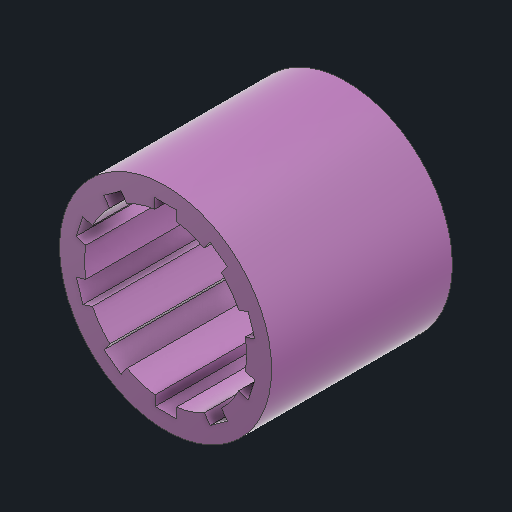
# Autodesk Inventor part: opona_CPY
Saved by Autodesk Inventor 2024 (Build 280153000, 153)
## iProperties
Created: 2024-05-24
Part Number: opona_CPY
Material: Generic
Document SubType Name: Modeling
Designer: Adam
Density: 1 g/cm^3
Appearance: Default
Author: Adam
Autodesk Inventor part; units mm, degrees
ref_plane "YZ Plane" through (0, 0, 0) normal (1, 0, 0) x (0, 1, 0)
ref_plane "XZ Plane" through (0, 0, 0) normal (0, 1, 0) x (-1, 0, 0)
ref_plane "XY Plane" through (0, 0, 0) normal (0, 0, 1) x (1, 0, 0)
sketch "Sketch1" plane through (0, 0, 0) normal (0, 0, 1) x (1, 0, 0)
  arc A0 (-12.7878, 2.3392) -> (-12.7811, -2.3759) centre (0, 0) ccw
  line L0 (-12.7811, -2.3759) -> (-14.3126, -2.8735)
  line L1 (-13.2567, -6.1232) -> (-14.3126, -2.8735)
  line L2 (-14.3126, -2.8735) -> (-13.2567, -6.1232)
  line L3 (-13.2567, -6.1232) -> (-11.7205, -5.624)
  line L4 (-13.2681, 6.088) -> (-14.324, 2.8383)
  line L5 (-14.324, 2.8383) -> (-12.7878, 2.3392)
  line L6 (-11.7366, 5.5904) -> (-13.2681, 6.088)
  arc A1 (-8.9706, 9.4089) -> (-11.7366, 5.5904) centre (0, 0) ccw
  line L7 (-7.1557, 12.7241) -> (-9.92, 10.7157)
  line L8 (-9.92, 10.7157) -> (-8.9706, 9.4089)
  line L9 (-6.2091, 11.4213) -> (-7.1557, 12.7241)
  arc A2 (-1.727, 12.8848) -> (-6.2091, 11.4213) centre (0, 0) ccw
  line L10 (1.69, 14.5) -> (-1.727, 14.5)
  line L11 (-1.727, 14.5) -> (-1.727, 12.8848)
  line L12 (1.69, 12.8897) -> (1.69, 14.5)
  arc A3 (6.1764, 11.4391) -> (1.69, 12.8897) centre (0, 0) ccw
  line L13 (9.8901, 10.7374) -> (7.1258, 12.7458)
  line L14 (7.1258, 12.7458) -> (6.1764, 11.4391)
  line L15 (8.9436, 9.4346) -> (9.8901, 10.7374)
  arc A4 (11.7205, 5.624) -> (8.9436, 9.4346) centre (0, 0) ccw
  line L16 (14.3126, 2.8735) -> (13.2567, 6.1232)
  line L17 (13.2567, 6.1232) -> (11.7205, 5.624)
  line L18 (12.7811, 2.3759) -> (14.3126, 2.8735)
  arc A5 (12.7878, -2.3392) -> (12.7811, 2.3759) centre (0, 0) ccw
  line L19 (13.2681, -6.088) -> (14.324, -2.8383)
  line L20 (14.324, -2.8383) -> (12.7878, -2.3392)
  line L21 (11.7366, -5.5904) -> (13.2681, -6.088)
  arc A6 (8.9706, -9.4089) -> (11.7366, -5.5904) centre (0, 0) ccw
  line L22 (7.1557, -12.7241) -> (9.92, -10.7157)
  line L23 (9.92, -10.7157) -> (8.9706, -9.4089)
  line L24 (6.2091, -11.4213) -> (7.1557, -12.7241)
  arc A7 (1.727, -12.8848) -> (6.2091, -11.4213) centre (0, 0) ccw
  line L25 (-1.69, -14.5) -> (1.727, -14.5)
  line L26 (1.727, -14.5) -> (1.727, -12.8848)
  line L27 (-1.69, -12.8897) -> (-1.69, -14.5)
  arc A8 (-6.1764, -11.4391) -> (-1.69, -12.8897) centre (0, 0) ccw
  line L28 (-9.8901, -10.7374) -> (-7.1258, -12.7458)
  line L29 (-7.1258, -12.7458) -> (-6.1764, -11.4391)
  line L30 (-8.9436, -9.4346) -> (-9.8901, -10.7374)
  arc A9 (-11.7205, -5.624) -> (-8.9436, -9.4346) centre (0, 0) ccw
  circle A10 centre (0, 0) radius 17
  point P0 (-8.9706, 9.4089)
  point P1 (-1.727, 12.8848)
  point P2 (6.1764, 11.4391)
  point P3 (12.7878, -2.3392)
  point P4 (-11.7205, -5.624)
  dimension "d2" = 360
  dimension "d3" = 34
  constraints: 62 end point, 20 point on circle, 11 centre point, 3 coincident, 101 other
  measures "d3" diameter of A10
extrude "Extrusion1" add sketch "Sketch1" along normal blind 29
body "Solid1"
